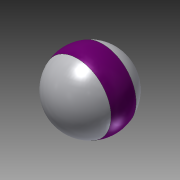
# Autodesk Inventor part: Pool_Ball_Stripe
Saved by Autodesk Inventor 2015 (Build 190159000, 159)
## iProperties
Created: 2016-12-24
Part Number: Pool_Ball_Stripe
Material: Generic
Document SubType Name: Modeling
Designer: Guy
Density: 1 g/cm^3
Appearance: Default
Author: Guy
Autodesk Inventor part; units mm, degrees
ref_plane "YZ Plane" through (0, 0, 0) normal (1, 0, 0) x (0, 1, 0)
ref_plane "XZ Plane" through (0, 0, 0) normal (0, 1, 0) x (-1, 0, 0)
ref_plane "XY Plane" through (0, 0, 0) normal (0, 0, 1) x (1, 0, 0)
sketch "Sketch1" plane through (0, 0, 0) normal (0, 0, 1) x (1, 0, 0)
  circle A0 centre (0, 0) radius 28.5
  line L0 (0, 28.5) -> (0, -28.5)
  dimension "d0" = 57
  constraints: 2 end point, 2 point on circle, 1 centre point, 1 coincident, 1 vertical
  measures "d0" diameter of A0
revolve "Revolution1" add sketch "Sketch1" angle 360 about axis through (0, 28.5, 0) along (0, -1, 0)
sketch "Sketch2" plane through (0, 0, 0) normal (1, 0, 0) x (0, 1, 0)
  line L0 (10, 26.6934) -> (10, -26.6934)
  line L1 (-10, 26.6934) -> (-10, -26.6934)
  circle A0 centre (0, 0) radius 28.505
  circle A1 centre (0, 0) radius 28.5 projected
  arc A2 (10, 26.688) -> (-10, 26.688) centre (0, 0) ccw
  arc A3 (-10, -26.688) -> (10, -26.688) centre (0, 0) ccw
  line L2 (-39.907, 0) -> (39.907, 0) projected
  dimension "d6" = 10
  dimension "d7" = 10
  dimension "d8" = 57.01
  constraints: 8 point on circle, 4 end point, 4 point on line, 3 centre point, 2 coincident, 2 vertical
  measures "d6" distance from line of point (0, 0) L0
  measures "d7" distance from line of L1 point (0, 0)
  measures "d8" diameter of A0
revolve "Revolution2" add sketch "Sketch2" angle 360 about axis through (0, -10, 0) along (0, 1, 0)
body "Solid1"
